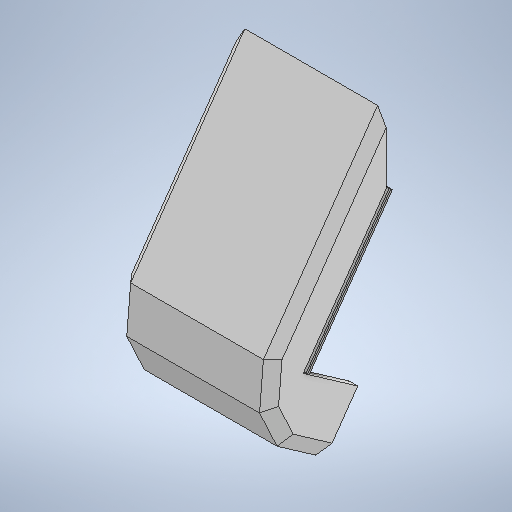
# Autodesk Inventor part: cameraholderlid v03
Saved by Autodesk Inventor 2025.2 (Build 292293000, 293)
## iProperties
Created: 2025-07-10
Part Number: cameraholderlid v03
Material: Generic
Document SubType Name: Modeling
Designer: mateo
Density: 1 g/cm^3
Appearance: Default
Author: mateo
Autodesk Inventor part; units mm, degrees
ref_plane "YZ Plane" through (0, 0, 0) normal (1, 0, 0) x (0, 1, 0)
ref_plane "XZ Plane" through (0, 0, 0) normal (0, 1, 0) x (-1, 0, 0)
ref_plane "XY Plane" through (0, 0, 0) normal (0, 0, 1) x (1, 0, 0)
sketch "Sketch1" plane through (0, 0, 0) normal (0, 0, 1) x (1, 0, 0)
  line L0 (40, -60) -> (-40, -60)
  line L1 (50, 50) -> (50, -50)
  line L2 (-50, -50) -> (-50, 50)
  line L3 (-40, 60) -> (40, 60)
  line L4 (50, -60) -> (50, 60)
  line L5 (50, 60) -> (-50, 60)
  line L6 (-50, 60) -> (-50, -60)
  line L7 (50, -60) -> (-50, -60)
  line L8 (-72, 82) -> (72, 82)
  line L9 (72, 82) -> (72, 0)
  line L10 (72, 0) -> (72, -82)
  line L11 (72, -82) -> (-72, -82)
  line L12 (-72, -82) -> (-72, 82)
  point P0 (0, 0)
  point P1 (0, 10)
  point P2 (0, 0)
  constraints: 26 end point, 3 perpendicular, 2 point on line, 1 collinear
extrude "Extrusion1" add sketch "Sketch1" along normal blind 5
sketch "Sketch2" plane through (0, 305, 5) normal (0, 0, 1) x (1, 0, 0)
  point P0 (0, 0)
  point P1 (-65, -305)
  point P2 (-65, -260)
  point P3 (-65, -350)
  point P4 (65, -305)
  point P5 (65, -260)
  point P6 (65, -350)
  point P7 (-20, -230)
  point P8 (20, -230)
  point P9 (-20, -380)
  point P10 (20, -380)
  dimension "d7" = 45
  dimension "d8" = 45
  dimension "d6" = 45
  dimension "d5" = 45
  measures "d7" distance of point (-65, -350) point (-65, -305)
  measures "d8" distance of point (-65, -305) point (-65, -260)
  measures "d6" distance of point (65, -305) point (65, -260)
  measures "d5" distance of point (65, -350) point (65, -305)
hole "Hole1" at (-65, 0, 5) at (-65, 45, 5) at (-65, -45, 5) at (65, 0, 5) at (65, 45, 5) at (65, -45, 5) at (-20, 75, 5) at (20, 75, 5) at (-20, -75, 5) at (20, -75, 5) direction (0, 0, -1) diameter 3.4587 depth 10.8 tip angle 118
move or copy body "Move Body1" bodies to move or copy 1 copy no translate (-2.5, -1.5, 0)
ref_plane "Work Plane1" through (-52.5, 58.5, 5) normal (0, -0.6427876, 0.7660444) x (1, 0, 0)
ref_plane "Work Plane2" through (47.5, -61.5, 5) normal (0, 0.5735764, 0.819152) x (-1, 0, 0)
sketch "Sketch6" plane through (47.5, -61.5, 5) normal (0, 0.5735764, 0.819152) x (-1, 0, 0)
  line L0 (102.232, 1.5875) -> (102.232, -110.9125)
  line L1 (-2.232, -110.9125) -> (-2.232, 1.5875)
  line L2 (-2.232, -110.9125) -> (102.232, -110.9125)
  line L3 (102.232, 1.5875) -> (102.232, 46.5875)
  line L4 (102.232, 46.5875) -> (-2.232, 46.5875)
  line L5 (-2.232, 46.5875) -> (-2.232, 1.5875)
  ellipse E0 centre (115, -12.2873) end of major axis (113.2706, -12.2873) minor radius 1.4166 projected
  ellipse E1 centre (-15, -12.2873) end of major axis (-16.7294, -12.2873) minor radius 1.4166 projected
  ellipse E2 centre (115, -49.1491) end of major axis (113.2706, -49.1491) minor radius 1.4166 projected
  ellipse E3 centre (-15, -49.1491) end of major axis (-16.7294, -49.1491) minor radius 1.4166 projected
  line L6 (102.232, 1.5875) -> (102.232, 46.5875)
  point P0 (47.5, -53.2457)
  dimension "d76" = 12.768
  dimension "d77" = 12.768
  dimension "d78" = 12.768
  dimension "d79" = 12.768
  constraints: 14 end point, 2 parallel, 2 perpendicular, 4 other
  measures "d76" distance from line of point (115, -12.287) L0
  measures "d77" distance from line of point (-15, -12.287) L1
  measures "d78" distance from line of L0 point (115, -49.149)
  measures "d79" distance from line of point (-15, -49.149) L1
extrude "Extrusion4" add sketch "Sketch6" along normal blind 70 contours L0 L2 L1 L5 L4 L3
sketch "Sketch8" plane through (47.5, -61.5, 5) normal (0, 0.5735764, 0.819152) x (-1, 0, 0)
  line L0 (0, -115.8875) -> (100, -115.8875) projected
  line L1 (0, -101.1661) -> (0, -2.8679) projected
  line L2 (96.232, -115.8875) -> (3.768, -115.8875)
  line L3 (102.232, 46.5875) -> (-2.232, 46.5875) projected
  line L4 (0, 46.5875) -> (100, 46.5875)
  line L5 (102.232, -110.9125) -> (102.232, -8.7172) projected
  line L6 (-2.232, -8.7172) -> (-2.232, -110.9125) projected
  line L7 (102.232, 0) -> (102.232, 46.5875) projected
  line L8 (96.232, 46.5875) -> (3.768, 46.5875)
  line L9 (3.768, 46.5875) -> (3.768, -115.8875)
  line L10 (3.768, -115.8875) -> (96.232, -115.8875)
  line L11 (96.232, -115.8875) -> (96.232, 46.5875)
  point P0 (47.5, -53.2457)
  point P1 (0, -8.7172)
  point P2 (96.232, -115.8875)
  point P3 (96.232, 46.5875)
  point P4 (3.768, 46.5875)
  point P5 (3.768, -115.8875)
  dimension "d42" = 6
  dimension "d43" = 6
  constraints: 12 end point, 2 horizontal, 2 parallel, 2 point on line, 1 perpendicular
  measures "d42" distance between parallel lines of L11 L5
  measures "d43" distance between parallel lines of L9 L6
extrude "Extrusion6" cut sketch "Sketch8" along normal blind 65
sketch "Sketch12" plane through (-54.732, -54.3593, 0) normal (-1, 0, 0) x (0, 0, 1)
  line L0 (0, 0) -> (0, 122.0413) projected
  line L1 (-1.2762, 123.8638) -> (0, 122.0413) projected
  line L2 (0, 122.0413) -> (-1.2762, 123.8638)
  line L3 (-1.2762, 123.8638) -> (-58.6698, 83.6763)
  line L4 (-58.6698, 83.6763) -> (0, -0.1129)
  line L5 (0, -0.1129) -> (0, 122.0413)
  point P0 (0, 54.3593)
  point P1 (0, 0)
  constraints: 8 end point, 2 perpendicular, 1 collinear, 1 vertical
extrude "Extrusion8" cut sketch "Sketch12" against normal through all
chamfer "Chamfer1" distance 6 angle 45 2 edges at (49.732, 0.5147, 47.0311) (-54.732, 0.5147, 47.0311)
sketch "Sketch15" plane through (47.5, -61.5, 5) normal (0, 0.5735764, 0.819152) x (-1, 0, 0)
  line L0 (96.232, -110.9125) -> (96.232, 46.5875) projected
  line L1 (3.768, -23.8125) -> (96.232, -23.8125)
  line L2 (96.232, -23.8125) -> (96.232, 11.2719)
  line L3 (3.768, 46.5875) -> (3.768, -110.9125) projected
  line L4 (3.768, 20.6375) -> (3.768, 46.5875)
  line L5 (3.768, 46.5875) -> (96.232, 46.5875)
  line L6 (96.232, 46.5875) -> (96.232, 11.2719)
  line L7 (102.232, 0) -> (102.232, 46.5875) projected
  line L8 (3.768, 46.5875) -> (3.768, -23.8125)
  point P0 (47.5, -53.2457)
  point P1 (96.6, -101.5469)
  point P2 (96.232, 46.5875)
  point P3 (2.1357, -101.5469)
  point P4 (3.768, -110.9125)
  point P5 (96.6, -100.9795)
  point P6 (2.1357, -100.9795)
  constraints: 12 end point, 1 parallel, 4 other
extrude "Extrusion11" add sketch "Sketch15" along normal blind 5 and the other way blind 3
ref_plane "Work Plane3" through (-54.732, -59.5119, 89.0621) normal (0, 0.819152, -0.5735764) x (1, 0, 0)
ref_plane "Work Plane7" through (-54.732, -84.9826, 28.6379) normal (0, 0.9786416, -0.205574) x (1, 0, 0)
sketch "Sketch28" plane through (-54.732, -84.9826, 28.6379) normal (0, 0.9786416, -0.205574) x (1, 0, 0)
  line L0 (104.464, -64.7463) -> (104.464, -63.1884) projected
  line L1 (104.464, -64.7463) -> (104.464, -63.1884)
  line L2 (98.464, -6.7829) -> (98.464, -69.7132) projected
  line L3 (104.464, -63.1884) -> (98.464, -69.7132)
  line L4 (6, -6.7829) -> (6, -69.7132) projected
  line L5 (98.464, -69.7132) -> (6, -69.7132)
  line L6 (0, -63.1884) -> (6, -69.7132) projected
  line L7 (6, -69.7132) -> (0, -63.1884)
  line L8 (0, -63.1884) -> (0, -64.7463)
  line L9 (0, -64.7463) -> (6, -70.2637)
  line L10 (6, -70.2637) -> (98.464, -70.2637)
  line L11 (98.464, -70.2637) -> (104.464, -64.7463)
  point P0 (54.732, 10.556)
  constraints: 16 end point, 3 equal length, 3 perpendicular, 1 vertical
extrude "Extrusion22" cut sketch "Sketch28" against normal through all
sketch "Sketch31" plane through (-54.732, -61.5, 5) normal (-1, 0, 0) x (0, 0, 1)
  line L0 (26.7215, -38.1622) -> (79.1472, -1.4534) projected
  line L1 (64.0809, -30.3145) -> (67.1645, -44.9941) projected
  line L2 (26.7215, -38.1622) -> (67.1645, -44.9941)
  line L3 (55.4773, -18.0272) -> (64.0809, -30.3145) projected
  line L4 (67.0706, -45.0138) -> (94.0685, -39.3427) projected
  line L5 (70.081, -44.3815) -> (67.0706, -45.0138)
  line L6 (70.081, -44.3815) -> (63.7303, -15.5115)
  line L7 (63.7303, -15.5115) -> (25.4, -18.0272)
  line L8 (25.4, -18.0272) -> (26.7215, -38.1622)
  point P0 (-5, 61.5)
  constraints: 10 end point, 1 collinear, 1 perpendicular, 1 point on line
extrude "Extrusion25" add sketch "Sketch31" against normal blind 6
sketch "Sketch32" plane through (49.732, -61.5, 5) normal (1, 0, 0) x (0, 0, -1)
  line L0 (-26.7215, -38.1622) -> (0, 0) projected
  line L1 (-26.7215, -38.1622) -> (-67.1645, -44.9941) projected
  line L2 (-26.7215, -38.1622) -> (-67.1645, -44.9941)
  line L3 (-64.0809, -30.3145) -> (-67.1645, -44.9941) projected
  line L4 (-67.1645, -44.9941) -> (-64.0809, -30.3145)
  line L5 (-55.4773, -18.0272) -> (-64.0809, -30.3145) projected
  line L6 (-64.0809, -30.3145) -> (-55.4773, -18.0272)
  line L7 (-55.4773, -18.0272) -> (-26.7215, -38.1622)
  line L8 (-67.1645, -44.9941) -> (-71.4375, -44.0965)
  line L9 (-94.0685, -39.3427) -> (-67.1656, -44.9939) projected
  line L10 (-71.4375, -44.0965) -> (-64.617, -11.6275)
  line L11 (-64.617, -11.6275) -> (-26.7215, -38.1622)
  point P0 (5, 61.5)
  constraints: 14 end point, 3 collinear, 3 perpendicular, 2 point on line
extrude "Extrusion26" add sketch "Sketch32" against normal blind 6
sketch "Sketch34" plane through (47.5, -58.6321, 9.0958) normal (0, 0.5735764, 0.819152) x (1, 0, 0)
  line L0 (-3.768, 15.858) -> (-3.768, -46.5875) projected
  line L1 (-96.232, -46.5875) -> (-96.232, 15.858) projected
  line L2 (-96.232, -46.5875) -> (-3.768, -46.5875) projected
  line L3 (-3.768, 23.8125) -> (-96.232, 23.8125) projected
  line L4 (-50, -46.5875) -> (-50, 23.8125)
  line L5 (-94, -46.5875) -> (-54, -46.5875)
  line L6 (-54, -46.5875) -> (-54, 3.4125)
  line L7 (-54, 3.4125) -> (-94, 3.4125)
  line L8 (-94, 3.4125) -> (-96.232, 3.4125)
  line L9 (-96.232, 3.4125) -> (-96.232, -46.5875)
  line L10 (-94, -46.5875) -> (-96.232, -46.5875)
  point P0 (-47.5, 53.2457)
  point P1 (-54, -46.5875)
  dimension "d100" = 92.464
  dimension "d101" = 70.4
  dimension "d112" = 50
  constraints: 14 end point, 4 perpendicular, 2 midpoint, 2 point on line, 1 horizontal, 1 parallel
  measures "d100" distance between parallel lines of L0 L1
  measures "d101" distance between parallel lines of L2 L3
  measures "d112" distance between parallel lines of L2 L7
extrude "Extrusion27" add sketch "Sketch34" along normal blind 16
sketch "Sketch35" plane through (47.5, -49.4549, 22.2022) normal (0, 0.5735764, 0.819152) x (1, 0, 0)
  circle A0 centre (-74.6125, -42.8625) radius 2
  circle A1 centre (-84.6125, -19.1625) radius 2
  line L0 (-74.6125, 141.2434) -> (-74.6125, 78.7138)
  circle A2 centre (-64.6125, -19.1625) radius 2
  line L1 (-220.5298, -133.1321) -> (71.3048, -56.0245)
  point P0 (-47.5, 53.2457)
  point P1 (-90.1769, -210.863)
  point P2 (-74.6125, -94.5783)
  point P3 (-74.6125, -94.5783)
  dimension "d115" = 4
  dimension "d117" = 4
  dimension "d121" = 50
  dimension "d122" = 20
  dimension "d123" = 23.7
  constraints: 4 end point, 3 centre point, 2 midpoint, 2 vertical alignment, 1 symmetric about line, 1 vertical, 1 other
  measures "d115" diameter of A0
  measures "d117" diameter of A1
  measures "d121" distance from line of L1 A0.centre
  measures "d122" distance of A2.centre A1.centre
  measures "d123" vertical distance of A0.centre A1.centre
extrude "Extrusion28" cut sketch "Sketch35" against normal blind 24.6695
sketch "Sketch36" plane through (-74.5, -83.5, 5) normal (0, 0, 1) x (1, 0, 0)
  line L0 (22, 22) -> (19.768, 22) projected
  line L1 (124.232, 0) -> (19.768, 0)
  line L2 (124.232, 13.701) -> (19.768, 13.701)
  line L3 (19.768, 13.701) -> (0, 13.701)
  line L4 (0, 164) -> (0, 0) projected
  line L5 (0, 13.701) -> (0, 0)
  line L6 (0, 0) -> (19.768, 0)
  line L7 (0, 0) -> (144, 0) projected
  line L8 (124.232, 13.701) -> (144, 13.701)
  line L9 (144, 0) -> (144, 164) projected
  line L10 (144, 13.701) -> (144, 0)
  line L11 (144, 0) -> (124.232, 0)
  point P0 (74.5, 83.5)
  point P1 (0, 13.701)
  constraints: 16 end point, 3 collinear, 2 point on line, 1 perpendicular
sketch "Sketch37" plane through (-49.732, -99.6622, 31.7215) normal (0, -0.819152, 0.5735764) x (1, 0, 0)
  line L0 (-5, 0) -> (99.464, 0) projected
  line L1 (0, 8) -> (0, 0)
  line L2 (94.464, 0) -> (94.4704, 0)
  line L3 (-5, 0) -> (99.464, 0) projected
  line L4 (94.4704, 0) -> (94.464, 0)
  line L5 (93.464, 0) -> (93.464, 5)
  line L6 (93.464, 0) -> (93.464, 5) projected
  line L7 (93.464, 5) -> (43.232, 5)
  line L8 (43.232, 5) -> (43.232, 21)
  line L9 (43.232, 5) -> (93.464, 5) projected
  line L10 (0, 8) -> (0, 0)
  line L11 (1, 21) -> (4.232, 21)
  line L12 (1, 8) -> (1, 21)
  line L13 (1, 29.2104) -> (1, 0) projected
  line L14 (1, -3) -> (1, 5) projected
  line L15 (0, 0) -> (0, -3)
  line L16 (93.464, -3) -> (93.464, 5) projected
  line L17 (1, -3) -> (93.464, -3)
  line L18 (93.464, -3) -> (93.464, 5)
  line L19 (1, 21) -> (43.232, 21)
  line L20 (-5, 0) -> (-5, 29.2104) projected
  line L21 (1, 21) -> (1, -3)
  line L22 (93.464, -3) -> (93.464, 5)
  line L23 (43.232, 5) -> (43.232, 21)
  point P0 (49.732, 31.1792)
  point P1 (0, 29.137)
  point P2 (1, 5)
  point P3 (0, 8)
  point P4 (93.464, 41.1414)
  point P5 (93.464, 65)
  point P6 (93.464, 35.1055)
  point P7 (1, 29.137)
  point P8 (1, 0)
  point P9 (1, 0)
  point P10 (93.464, 0)
  constraints: 30 end point, 4 vertical, 3 collinear, 3 horizontal, 3 perpendicular, 1 point on line, 10 other
extrude "Extrusion29" add sketch "Sketch37" along normal blind 15
sketch "Sketch38" plane through (-49.732, -111.9495, 40.3251) normal (0, -0.819152, 0.5735764) x (1, 0, 0)
  line L0 (3.232, 8) -> (3.232, 24) projected
  line L1 (43.232, 5) -> (43.232, 21) projected
  line L2 (3.232, 24) -> (43.232, 24)
  line L3 (43.232, 24) -> (43.232, 22.05)
  line L4 (43.232, 22.05) -> (3.232, 22.05)
  line L5 (3.232, 22.05) -> (3.232, 24)
  point P0 (49.732, 31.1792)
  point P1 (3.232, 22.05)
  dimension "d141" = 16
  constraints: 8 end point, 2 parallel, 1 horizontal, 1 perpendicular, 1 point on line
  measures "d141" distance of L0.start L0.end
extrude "Extrusion30" cut sketch "Sketch38" against normal blind 288.2125
extrude "Extrusion31" cut sketch "Sketch36" against normal blind 288.2125
sketch "Sketch40" plane through (47.5, -61.5, 5) normal (0, -0.5735764, -0.819152) x (-1, 0, 0)
  circle A0 centre (74.6125, -42.8625) radius 2 projected
  circle A1 centre (64.6125, -19.1625) radius 2 projected
  circle A2 centre (84.6125, -19.1625) radius 2 projected
  circle A3 centre (74.6125, -42.8625) radius 5.5
  circle A4 centre (84.6125, -19.1625) radius 5.5
  circle A5 centre (64.6125, -19.1625) radius 5.5
  point P0 (47.5, 53.2457)
  dimension "d136" = 11
  dimension "d137" = 11
  dimension "d138" = 11
  constraints: 3 centre point, 3 coincident
  measures "d136" diameter of A3
  measures "d137" diameter of A4
  measures "d138" diameter of A5
extrude "Extrusion32" cut sketch "Sketch40" along normal blind 3
fillet "Fillet1" radius 2 1 edges at (-2.5, -69.799, 5)
sketch "Sketch41" plane through (47.5, -58.6321, 9.0958) normal (0, 0.5735764, 0.819152) x (1, 0, 0)
  line L0 (-54, 3.4125) -> (-54, -61.5875) projected
  line L1 (22, -5.1598) -> (-122, -5.1598) projected
  line L2 (-3.768, -61.5875) -> (-54, -61.5875) projected
  circle A0 centre (-29.5, -43.75) radius 3.5
  circle A1 centre (-29.5, -15.75) radius 3.5
  point P0 (-47.5, 53.2457)
  dimension "d147" = 7
  dimension "d149" = 7
  dimension "d196" = 28
  constraints: 2 centre point
  measures "d147" diameter of A0
  measures "d149" diameter of A1
  measures "d196" distance of A1.centre A0.centre
extrude "Extrusion33" cut sketch "Sketch41" against normal through all
sketch "Sketch42" plane through (47.5, -61.5, 5) normal (0, -0.5735764, -0.819152) x (-1, 0, 0)
  line L0 (97.232, -46.5875) -> (2.768, -46.5875) projected
  arc A0 (33, -43.75) -> (33, -43.75) centre (29.5, -43.75) ccw projected
  circle A1 centre (29.5, -43.75) radius 3.5 projected
  circle A2 centre (29.5, -43.75) radius 7.5
  circle A3 centre (29.5, -15.75) radius 3.5 projected
  circle A4 centre (29.5, -15.75) radius 7.5
  point P0 (47.5, 53.2457)
  point P1 (2.768, -46.5875)
  point P2 (26, -43.75)
  point P3 (26, -43.75)
  dimension "d158" = 15
  dimension "d197" = 15
  constraints: 2 centre point, 2 coincident, 1 other
  measures "d158" diameter of A2
  measures "d197" diameter of A4
extrude "Extrusion34" cut sketch "Sketch42" along normal blind 3
sketch "Sketch44" plane through (47.5, -61.5, 5) normal (0, -0.5735764, -0.819152) x (-1, 0, 0)
  line L0 (102.232, -46.5875) -> (96.232, -46.5875) projected
  line L1 (96.232, 0) -> (96.232, -46.5875) projected
  line L2 (102.232, 0) -> (102.232, -46.5875) projected
  line L3 (100, 0) -> (102.232, 0) projected
  line L4 (96.232, 0) -> (100, 0) projected
  line L5 (100, 8.7172) -> (96.232, 8.7172) projected
  line L6 (96.232, 8.7172) -> (96.232, 0) projected
  line L7 (100, 8.7172) -> (100, 0) projected
  line L8 (96.232, 0) -> (96.232, 2.1006) projected
  line L9 (102.232, -46.5875) -> (96.232, -46.5875)
  line L10 (96.232, -46.5875) -> (96.232, 0)
  line L11 (96.232, 0) -> (102.232, 0)
  line L12 (102.232, 0) -> (102.232, -46.5875)
  line L13 (3.768, -46.5875) -> (3.768, 0) projected
  line L14 (0, 0) -> (3.768, 0) projected
  line L15 (-2.232, 0) -> (0, 0) projected
  line L16 (-2.232, -46.5875) -> (-2.232, 0) projected
  line L17 (3.768, 8.7172) -> (0, 8.7172) projected
  line L18 (0, 0) -> (0, 8.7172) projected
  line L19 (3.768, 0) -> (3.768, 8.7172) projected
  line L20 (2.768, -46.5875) -> (-2.232, -46.5875)
  line L21 (-2.232, -46.5875) -> (-2.232, 0)
  line L22 (-2.232, 0) -> (2.768, 0)
  line L23 (2.768, 0) -> (2.768, -46.5875)
  line L24 (96.232, 0) -> (100, 0) projected
  line L25 (102.232, -46.5875) -> (96.232, -46.5875)
  line L26 (96.232, -46.5875) -> (96.232, 0)
  line L27 (96.232, 0) -> (102.232, 0)
  line L28 (102.232, 0) -> (102.232, -46.5875)
  line L29 (-2.232, -46.5875) -> (-2.232, 0) projected
  line L30 (2.768, -46.5875) -> (-2.232, -46.5875)
  line L31 (-2.232, -46.5875) -> (-2.232, 0)
  line L32 (-2.232, 0) -> (2.768, 0)
  line L33 (2.768, 0) -> (2.768, -46.5875)
  line L34 (96.232, 0) -> (96.232, -46.5875) projected
  line L35 (102.232, 0) -> (102.232, -46.5875) projected
  line L36 (100, 0) -> (102.232, 0) projected
  line L37 (96.232, 0) -> (100, 0) projected
  line L38 (102.232, -46.5875) -> (96.232, -46.5875) projected
  line L39 (3.768, -46.5875) -> (-2.232, -46.5875) projected
  line L40 (100, 8.7172) -> (96.232, 8.7172) projected
  line L41 (96.232, 8.7172) -> (96.232, 0) projected
  line L42 (100, 8.7172) -> (100, 0) projected
  line L43 (3.768, -46.5875) -> (3.768, 0) projected
  line L44 (0, 0) -> (3.768, 0) projected
  line L45 (-2.232, 0) -> (0, 0) projected
  line L46 (-2.232, -46.5875) -> (-2.232, 0) projected
  line L47 (102.232, -46.5875) -> (96.232, -46.5875) projected
  line L48 (3.768, -46.5875) -> (-2.232, -46.5875) projected
  line L49 (3.768, 8.7172) -> (0, 8.7172) projected
  line L50 (0, 0) -> (0, 8.7172) projected
  line L51 (3.768, 0) -> (3.768, 8.7172) projected
  point P0 (47.5, 53.2457)
  point P1 (102.232, -46.5875)
  point P2 (2.768, 0)
  constraints: 32 end point, 8 parallel, 4 horizontal, 4 perpendicular
extrude "Extrusion35" add sketch "Sketch44" along normal blind 3 contours L0 L1 L4 L3 L2 | L39 L23 L14 L13 | L20 L16 L15 L14 L23
ref_plane "Work Plane8" through (44.732, -106.4941, 72.1645) normal (0, -0.9860303, -0.166566) x (1, 0, 0)
sketch "Sketch45" plane through (44.732, -106.4941, 72.1645) normal (0, -0.9860303, -0.166566) x (1, 0, 0)
  line L0 (-99.464, -41.016) -> (-99.464, 0) projected
  line L1 (-99.464, -41.016) -> (5, -41.016) projected
  line L2 (5, 0) -> (5, -41.016) projected
  line L3 (-1, -33.9952) -> (-1, 0) projected
  line L4 (-1, -41.016) -> (5, -41.016) projected
  line L5 (-99.464, 0) -> (-93.464, 0)
  line L6 (-99.464, -41.016) -> (-99.464, 0)
  line L7 (5, 0) -> (5, -41.016) projected
  line L8 (0, 0) -> (5, 0)
  line L9 (5, 0) -> (5, -41.016)
  line L10 (-1, -41.016) -> (-1, -33.9952) projected
  line L11 (5, -72.8496) -> (5, -43.1525) projected
  line L12 (5, -43.1525) -> (-99.464, -43.1525) projected
  line L13 (5, -43.1525) -> (-1, -43.1525)
  line L14 (-1, -43.1525) -> (-1, 0)
  line L15 (5, 0) -> (5, -43.1525)
  line L16 (5, -43.1525) -> (-99.464, -43.1525) projected
  line L17 (-99.464, -41.016) -> (-99.464, -43.1525)
  line L18 (-99.464, -43.1525) -> (-93.464, -43.1525)
  line L19 (-93.464, -43.1525) -> (-93.464, -41.016)
  line L20 (-93.464, 0) -> (-99.464, 0)
  line L21 (-99.464, 0) -> (-99.464, -43.1525)
  line L22 (-99.464, -43.1525) -> (-93.464, -43.1525)
  line L23 (-93.464, 0) -> (-93.464, -43.1525)
  line L24 (-93.464, -98.7163) -> (-93.464, 15.8051) projected
  line L25 (5, 0) -> (-1, 0) projected
  point P0 (-44.732, -88.8947)
  point P1 (-94.464, -0.1031)
  point P2 (-94.464, -41.016)
  point P3 (-93.464, -0.1031)
  point P4 (5, -41.016)
  point P5 (-1, -41.016)
  point P6 (-93.464, -41.016)
  point P7 (-99.464, -41.016)
  constraints: 28 end point, 7 collinear, 3 horizontal, 1 perpendicular, 1 vertical
extrude "Extrusion37" add sketch "Sketch45" along normal blind 15 contours L0 L5 L23 L1 | L1 L19 L12 L17 | L1 L15 L12 L14
sketch "Sketch47" plane through (49.732, -66.7303, 5) normal (1, 0, 0) x (0, 0, -1)
  line L0 (-67.0629, -39.7466) -> (-67.0706, -39.7835) projected
  line L1 (-67.0706, -39.7835) -> (-27.0245, -48.1956)
  line L2 (-64.6661, -54.5542) -> (-22.1163, -47.3665) projected
  line L3 (-27.0245, -48.1956) -> (-64.578, -54.5394)
  line L4 (-67.1645, -39.7638) -> (-94.0685, -34.1123) projected
  line L5 (-64.578, -54.5394) -> (-64.6661, -54.5542)
  line L6 (-67.1645, -39.7638) -> (-64.6661, -54.5542) projected
  line L7 (-67.1645, -39.7638) -> (-67.0706, -39.7835)
  point P0 (5, 66.7303)
  point P1 (-32.8677, -46.9399)
  point P2 (-24.223, -47.7224)
  point P3 (-63.9955, -25.144)
  constraints: 8 end point, 2 collinear, 1 point on line
extrude "Extrusion38" cut sketch "Sketch47" against normal blind 120
sketch "Sketch49" plane through (-48.732, -54.3593, 0) normal (-1, 0, 0) x (0, 0, 1)
  line L0 (0, 8.7172) -> (44.4209, -54.7224) projected
  line L1 (0, 8.7172) -> (0, -5.2303)
  line L2 (1.3377, -7.1407) -> (-11.1157, 10.6446) projected
  line L3 (-11.1157, 10.6446) -> (-4.3813, 15.3601)
  line L4 (-4.3813, 15.3601) -> (0, 8.7172)
  line L5 (0, 8.7172) -> (-4.5625, 15.2332) projected
  line L6 (-11.1157, 10.6446) -> (0, -5.2303)
  point P0 (0, 54.3593)
  constraints: 8 end point, 3 point on line, 2 perpendicular, 1 vertical
extrude "Extrusion40" cut sketch "Sketch49" against normal through all contours L1 L2 L3 L5
sketch "Sketch50" plane through (-48.732, -55.8368, 7.1384) normal (0, 0.819152, -0.5735764) x (1, 0, 0)
  line L0 (42.232, -16) -> (0, -16) projected
  line L1 (9.0575, -16) -> (7.9375, -16)
  arc A0 (34.925, -16) -> (9.0575, -16) centre (21.9913, -30.5193) ccw
  line L2 (34.925, -16) -> (9.0575, -16)
  point P0 (48.732, -26.1792)
  point P1 (33.6195, -16)
  point P2 (9.0575, -16)
  constraints: 4 end point, 2 point on circle, 2 point on line, 1 centre point
extrude "Extrusion41" cut sketch "Sketch50" against normal blind 18.575
sketch "Sketch52" plane through (-54.732, -66.7303, 5) normal (-1, 0, 0) x (0, 0, 1)
  line L0 (26.7215, -32.9319) -> (24.223, -47.7224) projected
  line L1 (27.0245, -48.1956) -> (94.0685, -34.1123) projected
  line L2 (24.223, -47.7224) -> (27.0245, -48.1956) projected
  line L3 (32.8677, -46.9399) -> (26.0097, -37.1457) projected
  line L4 (26.0097, -37.1457) -> (32.8677, -46.9399)
  line L5 (27.0245, -48.1956) -> (24.223, -47.7224)
  line L6 (26.0097, -37.1457) -> (24.223, -47.7224)
  line L7 (32.8677, -46.9399) -> (32.9391, -47.042)
  line L8 (32.9391, -47.042) -> (27.0245, -48.1956)
  point P0 (-5, 66.7303)
  point P1 (32.8849, -46.9646)
  constraints: 10 end point, 2 collinear, 1 perpendicular, 1 point on line
extrude "Extrusion43" cut sketch "Sketch52" against normal through all contours L3 L7 L1 L2 L0
sketch "Sketch53" plane through (-54.732, -66.7303, 5) normal (-1, 0, 0) x (0, 0, 1)
  line L0 (0, 116.8109) -> (85.4767, -5.2624) projected
  line L1 (12.7, 98.6735) -> (85.4767, -5.2624)
  line L2 (12.7, 81.631) -> (12.7, 130.812)
  line L3 (12.7, 130.812) -> (12.7, 81.631)
  line L4 (12.7, 81.631) -> (12.7, 61.9125)
  line L5 (12.7, 61.9125) -> (102.0312, -65.6657)
  line L6 (12.7, 130.812) -> (-12.7, 180.975)
  line L7 (-12.7, 180.975) -> (-12.7, -92.075)
  line L8 (-12.7, -92.075) -> (102.0312, -65.6657)
  point P0 (-5, 66.7303)
  point P1 (87.7509, -8.5103)
  dimension "d233" = 145
  constraints: 16 end point, 2 point on line, 2 vertical, 1 collinear
  measures "d233" angle of L5 L4
extrude "Extrusion44" cut sketch "Sketch53" against normal through all
sketch "Sketch56" plane through (-54.732, -66.7303, 5) normal (-1, 0, 0) x (0, 0, 1)
  line L0 (24.264, -34.6526) -> (22.1163, -47.3665) projected
  line L1 (24.223, -47.7224) -> (26.0097, -37.1457) projected
  line L2 (24.264, -34.6526) -> (26.0097, -37.1457)
  line L3 (26.0097, -37.1457) -> (24.223, -47.7224)
  line L4 (24.223, -47.7224) -> (21.9676, -47.3414)
  line L5 (21.9676, -47.3414) -> (24.264, -34.6526)
  point P0 (-5, 66.7303)
  constraints: 8 end point, 1 collinear, 1 perpendicular
extrude "Extrusion46" cut sketch "Sketch56" against normal through all contours L2 L1 L4 L0
sketch "Sketch59" plane through (69.5, 80.5, 0) normal (0, 0, -1) x (-1, 0, 0)
  line L0 (124.232, -148.2248) -> (124.232, -65.5994) projected
  line L1 (124.232, -131.7625) -> (22.225, -131.7625)
  line L2 (22.225, -144.4625) -> (124.232, -144.4625)
  line L3 (124.232, -144.4625) -> (124.232, -131.7625)
  line L4 (22.225, -144.4625) -> (19.05, -144.4625)
  line L5 (19.05, -144.4625) -> (19.05, -131.7625)
  line L6 (19.05, -131.7625) -> (22.225, -131.7625)
  point P0 (69.5, -80.5)
  point P1 (22.225, -131.7625)
  constraints: 12 end point, 2 horizontal, 2 parallel, 1 perpendicular, 1 point on line
extrude "Extrusion48" add sketch "Sketch59" against normal blind 1
sketch "Sketch60" plane through (-74.5, 80.5, 0) normal (-1, 0, 0) x (0, 0, 1)
  line L0 (17.4625, 4.7625) -> (-19.05, 4.7625)
  line L1 (-19.05, 4.7625) -> (-19.05, -168.275)
  line L2 (-19.05, -168.275) -> (17.4625, -168.275)
  line L3 (17.4625, -168.275) -> (17.4625, 4.7625)
  point P0 (0, -80.5)
  constraints: 8 end point, 2 parallel, 1 horizontal, 1 perpendicular
extrude "Extrusion50" cut sketch "Sketch60" against normal through all
sketch "Sketch61" plane through (49.732, -4.8178, 17.7) normal (1, 0, 0) x (0, 0, -1)
  line L0 (-49.1752, -70.2295) -> (-66.4472, -58.1355) projected
  line L1 (-51.9844, -68.2625) -> (-49.1752, -70.2295)
  line L2 (-53.6682, -76.6461) -> (-51.917, -68.3097) projected
  line L3 (-54.6484, -78.4401) -> (-51.917, -68.3097)
  line L4 (-54.6484, -78.4401) -> (-47.625, -71.4375)
  line L5 (-49.1752, -70.2295) -> (-47.625, -71.4375)
  line L6 (-49.1752, -70.2295) -> (-51.917, -68.3097)
  point P0 (17.7, 4.8178)
  constraints: 10 end point, 2 collinear, 1 point on line
extrude "Extrusion51" cut sketch "Sketch61" against normal blind 149.7
sketch "Sketch62" plane through (-48.732, -62.3798, 84.9664) normal (0, -0.819152, 0.5735764) x (1, 0, 0)
  line L0 (-6, -22.0852) -> (0, -22.0852) projected
  line L1 (-2, -22.0852) -> (-2, -27.0852)
  line L2 (-4, -27.0852) -> (-4, -22.0852)
  line L3 (-6, -22.0852) -> (-6, -29.1506)
  line L4 (-1, -28.5852) -> (-5, -28.5852)
  line L5 (-5, -28.5852) -> (-5, -27.0852)
  line L6 (-1, -28.5852) -> (-1, -27.0852)
  line L7 (0, -22.0852) -> (0, -28.5852)
  line L8 (-4, -22.0852) -> (-4, -22.0852)
  line L9 (-6, -22.0852) -> (0, -22.0852) projected
  line L10 (-2, -22.0852) -> (-2, -22.0852)
  line L11 (-5, -27.0852) -> (-4, -27.0852)
  line L12 (-2, -27.0852) -> (-1, -27.0852)
  line L13 (-6, -22.0852) -> (-6, -1) projected
  line L14 (-6, -11.5426) -> (46.232, -11.5426)
  line L15 (46.232, -11.5426) -> (46.232, 19.05)
  line L16 (46.232, 19.05) -> (46.232, -31.75)
  line L17 (94.464, -22.0852) -> (94.464, -27.0852)
  line L18 (96.464, -27.0852) -> (96.464, -22.0852)
  line L19 (93.464, -28.5852) -> (97.464, -28.5852)
  line L20 (97.464, -28.5852) -> (97.464, -27.0852)
  line L21 (93.464, -28.5852) -> (93.464, -27.0852)
  line L22 (97.464, -27.0852) -> (96.464, -27.0852)
  line L23 (94.464, -27.0852) -> (93.464, -27.0852)
  line L24 (94.464, -22.0852) -> (94.464, -22.0432)
  line L25 (94.464, -22.0432) -> (96.464, -22.0432)
  line L26 (98.464, -22.0852) -> (92.464, -22.0852) projected
  line L27 (96.464, -22.0432) -> (96.464, -22.0852)
  point P0 (48.732, -33.8208)
  point P1 (0, -25.3352)
  point P2 (-2, -22.0852)
  dimension "d226" = 2
  dimension "d227" = 1.5
  dimension "d228" = 1
  dimension "d229" = 1
  dimension "d230" = 2
  dimension "d236" = 52.232
  constraints: 48 end point, 8 symmetric about line, 5 vertical, 4 parallel, 4 point on line, 3 horizontal, 3 perpendicular, 2 midpoint, 1 collinear
  measures "d226" distance between parallel lines of L2 L3
  measures "d227" distance of L4.end L5.end
  measures "d228" distance between parallel lines of L7 L6
  measures "d229" distance between parallel lines of L3 L5
  measures "d230" distance from line of point (0, -25.335) L1
  measures "d236" distance of L14.start L14.end
extrude "Extrusion52" add sketch "Sketch62" against normal up to surface (85.7344 mm away)
sketch "Sketch63" plane through (-48.732, -62.3798, 84.9664) normal (0, -0.819152, 0.5735764) x (1, 0, 0)
  line L0 (-6, -22.0852) -> (-6, -1) projected
  line L1 (-6, -1) -> (-6, -22.0852) projected
  line L2 (-6, -22.0852) -> (-6, -1)
  line L3 (-6, -1) -> (0, 5) projected
  line L4 (-6, -1) -> (0, 5)
  line L5 (0, 5) -> (92.464, 5)
  line L6 (92.464, 5) -> (98.464, -1)
  line L7 (98.464, -1) -> (98.464, -22.0852)
  line L8 (92.464, 0) -> (92.464, -22.0852) projected
  line L9 (92.464, -22.0852) -> (92.464, 0)
  line L10 (92.464, 0) -> (0, 0)
  line L11 (0, 0) -> (0, -21.358)
  line L12 (-2, -22.0852) -> (0, -22.0852) projected
  line L13 (0, -22.0852) -> (0, -21.358)
  line L14 (0, -22.0852) -> (0, 0) projected
  line L15 (-6, -22.0852) -> (-4, -22.0852) projected
  line L16 (-4, -27.0852) -> (-4, -22.0852) projected
  line L17 (-4, -22.0852) -> (-4, -27.0852)
  line L18 (-5, -27.0852) -> (-5, -28.5852) projected
  line L19 (0, -22.0852) -> (0, 0) projected
  line L20 (0, 0) -> (92.464, 0) projected
  line L21 (92.464, 0) -> (92.464, -22.0852) projected
  line L22 (98.464, -22.0852) -> (96.464, -22.0852) projected
  line L23 (98.464, -22.0852) -> (98.464, -1) projected
  line L24 (92.464, 5) -> (98.464, -1) projected
  line L25 (0, 5) -> (92.464, 5) projected
  line L26 (-6, -1) -> (0, 5) projected
  line L27 (-6, -22.0852) -> (-6, -1) projected
  line L28 (-6, -22.0852) -> (-4, -22.0852) projected
  line L29 (-4, -22.0852) -> (-4, -27.0852) projected
  line L30 (-4, -27.0852) -> (-5, -27.0852) projected
  line L31 (-5, -27.0852) -> (-5, -28.5852) projected
  line L32 (-5, -28.5852) -> (-1, -28.5852) projected
  line L33 (-1, -28.5852) -> (-1, -27.0852) projected
  line L34 (-1, -27.0852) -> (-2, -27.0852) projected
  line L35 (-2, -27.0852) -> (-2, -22.0852) projected
  line L36 (-2, -22.0852) -> (0, -22.0852) projected
  line L37 (-4, -27.0852) -> (-5, -27.0852) projected
  line L38 (-4, -27.0852) -> (-5, -27.0852)
  line L39 (-5, -28.5852) -> (-5, -27.0852) projected
  line L40 (-5, -27.0852) -> (-5, -28.5852)
  line L41 (-5, -28.5852) -> (-1, -28.5852) projected
  line L42 (-5, -28.5852) -> (-1, -28.5852)
  line L43 (-1, -28.5852) -> (-1, -27.0852)
  line L44 (-2, -27.0852) -> (-2, -22.0852)
  line L45 (0, -22.0852) -> (-2, -22.0852)
  line L46 (-4, -22.0852) -> (-6, -22.0852)
  line L47 (94.464, -22.0852) -> (92.464, -22.0852) projected
  line L48 (94.464, -22.0852) -> (94.464, -27.0852) projected
  line L49 (94.464, -27.0852) -> (93.464, -27.0852) projected
  line L50 (93.464, -27.0852) -> (93.464, -28.5852) projected
  line L51 (93.464, -28.5852) -> (97.464, -28.5852) projected
  line L52 (97.464, -28.5852) -> (97.464, -27.0852) projected
  line L53 (97.464, -27.0852) -> (96.464, -27.0852) projected
  line L54 (96.464, -27.0852) -> (96.464, -22.0852) projected
  line L55 (96.464, -22.0852) -> (96.464, -27.0852)
  line L56 (97.464, -27.0852) -> (97.464, -28.5852)
  line L57 (96.464, -27.0852) -> (97.464, -27.0852)
  line L58 (97.464, -28.5852) -> (93.464, -28.5852)
  line L59 (93.464, -27.0852) -> (94.464, -27.0852)
  line L60 (94.464, -27.0852) -> (94.464, -22.0852)
  line L61 (93.464, -28.5852) -> (93.464, -27.0852)
  point P0 (48.732, -33.8208)
  point P1 (-2, -22.0852)
  point P2 (-4, -27.0852)
  point P3 (-5, -27.0852)
  point P4 (-5, -28.5852)
  constraints: 49 end point, 9 collinear, 7 perpendicular, 1 parallel
extrude "Extrusion53" add sketch "Sketch63" along normal blind 15.03
ref_plane "Work Plane9" through (-53.732, -91.0874, 70.1716) normal (0, -0.9961947, 0.0871557) x (1, 0, 0)
sketch "Sketch65" plane through (-53.732, -91.0874, 70.1716) normal (0, -0.9961947, 0.0871557) x (1, 0, 0)
  line L0 (5, 5.6292) -> (5, 24.7555) projected
  line L1 (3, 5.6292) -> (5, 5.6292) projected
  line L2 (-1, 23.8895) -> (-1, 5.6292) projected
  line L3 (-1, 5.6292) -> (1, 5.6292) projected
  line L4 (99.464, 5.6292) -> (99.464, 1.299) projected
  line L5 (99.464, 1.299) -> (98.464, 1.299) projected
  line L6 (98.464, 1.299) -> (98.464, 0) projected
  line L7 (98.464, 0) -> (102.464, 0) projected
  line L8 (102.464, 0) -> (102.464, 1.299) projected
  line L9 (102.464, 1.299) -> (101.464, 1.299) projected
  line L10 (101.464, 1.299) -> (101.464, 5.6292) projected
  line L11 (101.464, 5.6292) -> (103.464, 5.6292) projected
  line L12 (103.464, 5.6292) -> (103.464, 23.8895) projected
  line L13 (103.464, 23.8895) -> (97.464, 29.0857) projected
  line L14 (97.464, 29.0857) -> (5, 29.0857) projected
  line L15 (5, 29.0857) -> (-1, 23.8895) projected
  line L16 (-1, 23.8895) -> (-1, 5.6292) projected
  line L17 (-1, 5.6292) -> (1, 5.6292) projected
  line L18 (1, 5.6292) -> (1, 1.299) projected
  line L19 (1, 1.299) -> (0, 1.299) projected
  line L20 (0, 1.299) -> (0, 0) projected
  line L21 (0, 0) -> (4, 0) projected
  line L22 (4, 0) -> (4, 1.299) projected
  line L23 (4, 1.299) -> (3, 1.299) projected
  line L24 (3, 1.299) -> (3, 5.6292) projected
  line L25 (3, 5.6292) -> (5, 5.6292) projected
  line L26 (5, 5.6292) -> (5, 24.7555) projected
  line L27 (5, 24.7555) -> (97.464, 24.7555) projected
  line L28 (97.464, 24.7555) -> (97.464, 5.6292) projected
  line L29 (97.464, 5.6292) -> (99.464, 5.6292) projected
  line L30 (-1, 5.6292) -> (5, 5.6292)
  line L31 (5, 5.6292) -> (5, 24.7555)
  line L32 (5, 24.7555) -> (97.464, 24.7555)
  line L33 (97.464, 24.7555) -> (97.464, 5.6292)
  line L34 (97.464, 5.6292) -> (103.464, 5.6292)
  line L35 (103.464, 23.8895) -> (103.464, -41.5491) projected
  line L36 (103.464, 5.6292) -> (103.464, 23.8895)
  line L37 (103.464, 23.8895) -> (97.464, 29.0857)
  line L38 (97.464, 29.0857) -> (5, 29.0857)
  line L39 (5, 29.0857) -> (-1, 23.8895)
  line L40 (-1, 23.8895) -> (-1, 5.6292)
  point P0 (53.732, -61.9658)
  constraints: 20 end point, 5 collinear, 2 perpendicular, 1 horizontal, 1 vertical
extrude "Extrusion55" add sketch "Sketch65" along normal mid plane 35 contours L1 L30 L3 L2 L15 L14 L13 L12 L11 L34 L29 L28 L27 L0
sketch "Sketch67" plane through (-53.732, -73.654, 68.6464) normal (0, 0.9961947, -0.0871557) x (1, 0, 0)
  line L0 (97.464, -28.6772) -> (103.464, -21.749) projected
  line L1 (103.464, -23.8895) -> (103.464, -21.749) projected
  line L2 (103.464, -23.8895) -> (103.464, -21.749)
  line L3 (97.464, 40.6374) -> (97.464, -28.6772) projected
  line L4 (103.464, -21.749) -> (97.464, -28.6772)
  line L5 (5, 40.6374) -> (5, -28.6772) projected
  line L6 (97.464, -28.6772) -> (5, -28.6772)
  line L7 (-1, -21.749) -> (-1, -23.8895) projected
  line L8 (5, -28.6772) -> (-1, -21.749)
  line L9 (-1, -21.749) -> (-1, -23.8895)
  line L10 (-1, -23.8895) -> (5, -29.0857)
  line L11 (5, -29.0857) -> (97.464, -29.0857)
  line L12 (97.464, -29.0857) -> (103.464, -23.8895)
  point P0 (53.732, 61.9658)
  constraints: 16 end point, 4 equal length, 3 perpendicular
extrude "Extrusion56" cut sketch "Sketch67" against normal through all
ref_plane "Work Plane10" through (-54.732, -108.0302, 77.3046) normal (0, -0.9063078, -0.4226183) x (1, 0, 0)
sketch "Sketch68" plane through (-54.732, -108.0302, 77.3046) normal (0, -0.9063078, -0.4226183) x (1, 0, 0)
  line L0 (0, 13.9602) -> (0, 0) projected
  line L1 (6, 19.9602) -> (0, 13.9602) projected
  line L2 (0, 13.9602) -> (0, 0) projected
  line L3 (0, 0) -> (6, 0) projected
  line L4 (6, 0) -> (6, 16.5639) projected
  line L5 (6, 16.5639) -> (98.464, 16.5639) projected
  line L6 (98.464, 16.5639) -> (98.464, 0) projected
  line L7 (98.464, 0) -> (104.464, 0) projected
  line L8 (104.464, 0) -> (104.464, 13.9602) projected
  line L9 (104.464, 13.9602) -> (98.464, 19.9602) projected
  line L10 (98.464, 19.9602) -> (6, 19.9602) projected
  line L11 (0, 0) -> (6, 0) projected
  line L12 (6, 0) -> (0, 0)
  line L13 (0, 0) -> (0, 13.9602)
  line L14 (0, 13.9602) -> (6, 19.9602)
  line L15 (6, 19.9602) -> (98.464, 19.9602)
  line L16 (98.464, 19.9602) -> (104.464, 13.9602)
  line L17 (104.464, 0) -> (104.464, 13.9602) projected
  line L18 (104.464, 13.9602) -> (104.464, 0)
  line L19 (104.464, 0) -> (98.464, 0)
  line L20 (98.464, 0) -> (98.464, 16.5639)
  line L21 (98.464, 16.5639) -> (6, 16.5639)
  line L22 (6, 16.5639) -> (6, 0)
  line L23 (6, 16.5639) -> (98.464, 16.5639)
  line L24 (98.464, 16.5639) -> (98.464, 14.5516)
  line L25 (98.464, 14.5516) -> (6, 14.5516)
  line L26 (6, 14.5516) -> (6, 16.5639)
  point P0 (54.732, -115.7173)
  point P1 (6, 14.5516)
  point P2 (98.464, 14.5516)
  constraints: 29 end point, 6 equal length, 3 perpendicular, 2 horizontal, 2 point on line
extrude "Extrusion57" add sketch "Sketch68" along normal mid plane 30
ref_plane "Work Plane11" through (-54.732, -121.6249, 70.9653) normal (0, -0.5735764, -0.819152) x (1, 0, 0)
sketch "Sketch69" plane through (-54.732, -94.4356, 83.6438) normal (0, 0.9063078, 0.4226183) x (1, 0, 0)
  line L0 (104.464, 3.5398) -> (104.464, -9.9534) projected
  line L1 (104.464, -13.9602) -> (104.464, -9.9534) projected
  line L2 (104.464, -9.9534) -> (104.464, -13.9602)
  line L3 (98.464, -19.9602) -> (104.464, -13.9602) projected
  line L4 (104.464, -13.9602) -> (98.464, -19.9602)
  line L5 (98.464, -19.9602) -> (6, -19.9602)
  line L6 (6, -17.9534) -> (98.464, -17.9534) projected
  line L7 (6, -19.9602) -> (0, -13.9602)
  line L8 (0, -13.9602) -> (0, -9.9534)
  line L9 (0, -9.9534) -> (6, -17.9534) projected
  line L10 (0, -9.9534) -> (6, -17.9534)
  line L11 (6, -17.9534) -> (98.464, -17.9534)
  line L12 (98.464, -17.9534) -> (104.464, -9.9534) projected
  line L13 (98.464, -17.9534) -> (104.464, -9.9534)
  point P0 (54.732, 115.7173)
  constraints: 16 end point, 7 equal length, 1 perpendicular
extrude "Extrusion58" cut sketch "Sketch69" against normal through all
sketch "Sketch70" plane through (-54.732, -121.6249, 70.9653) normal (0, -0.5735764, -0.819152) x (1, 0, 0)
  line L0 (6, 15.5481) -> (0, 8.6199) projected
  line L1 (0, 8.6199) -> (0, 0) projected
  line L2 (0, 0) -> (6, 0) projected
  line L3 (6, 0) -> (6, 12.6021) projected
  line L4 (98.464, 12.6021) -> (98.464, 0) projected
  line L5 (98.464, 0) -> (104.464, 0) projected
  line L6 (104.464, 0) -> (104.464, 8.6199) projected
  line L7 (104.464, 8.6199) -> (98.464, 15.5481) projected
  line L8 (98.464, 15.5481) -> (6, 15.5481) projected
  line L9 (6, 12.6021) -> (98.464, 12.6021) projected
  line L10 (6, 12.6021) -> (98.464, 12.6021)
  line L11 (98.464, 12.6021) -> (98.464, 9.5481)
  line L12 (98.464, 9.5481) -> (6, 9.5481)
  line L13 (6, 9.5481) -> (6, 12.6021)
  point P0 (54.732, -140.3333)
  point P1 (6, 9.5481)
  dimension "d259" = 6
  constraints: 8 end point, 2 parallel, 1 horizontal, 1 perpendicular, 1 point on line
  measures "d259" distance between parallel lines of L12 L8
extrude "Extrusion59" add sketch "Sketch70" along normal mid plane 20
sketch "Sketch71" plane through (-54.732, -115.8891, 79.1568) normal (0, 0.5735764, 0.819152) x (1, 0, 0)
  line L0 (98.464, -14.9573) -> (104.464, -5.7197) projected
  line L1 (6, -14.9573) -> (98.464, -14.9573) projected
  line L2 (0, -5.7197) -> (6, -14.9573) projected
  line L3 (0, -5.7197) -> (0, -8.6199) projected
  line L4 (0, -8.6199) -> (6, -15.5481) projected
  line L5 (6, -15.5481) -> (98.464, -15.5481) projected
  line L6 (98.464, -15.5481) -> (104.464, -8.6199) projected
  line L7 (104.464, -8.6199) -> (104.464, -5.7197) projected
  point P0 (54.732, 140.3333)
extrude "Extrusion60" cut sketch "Sketch71" against normal through all
sketch "Sketch72" plane through (-54.732, -4.8178, 17.7) normal (-1, 0, 0) x (0, 0, 1)
  line L0 (45.0738, -122.5428) -> (48.3544, -127.228) projected
  line L1 (45.0738, -122.5428) -> (30.4648, -101.6789)
  line L2 (57.7961, -82.5414) -> (59.6046, -103.2124) projected
  line L3 (57.7961, -82.5414) -> (30.4648, -101.6789)
  line L4 (59.6046, -103.2124) -> (53.2653, -116.807) projected
  line L5 (57.7961, -82.5414) -> (59.6046, -103.2124)
  line L6 (59.6046, -103.2124) -> (53.2653, -116.807) projected
  line L7 (53.2653, -116.807) -> (45.0738, -122.5428) projected
  point P0 (-17.7, 4.8178)
  constraints: 6 end point, 1 collinear, 1 perpendicular
extrude "Extrusion61" add sketch "Sketch72" against normal blind 6
sketch "Sketch73" plane through (49.732, -4.8178, 17.7) normal (1, 0, 0) x (0, 0, -1)
  line L0 (-50.5503, -130.3641) -> (-30.4648, -101.6789) projected
  line L1 (-30.4648, -101.6789) -> (-57.7961, -82.5414) projected
  line L2 (-59.6046, -103.2124) -> (-53.2653, -116.807) projected
  line L3 (-53.2653, -116.807) -> (-45.0738, -122.5428) projected
  line L4 (-57.7961, -82.5414) -> (-59.6046, -103.2124) projected
  point P0 (17.7, 4.8178)
  point P1 (-52.302, -132.8658)
extrude "Extrusion62" add sketch "Sketch73" against normal blind 6
sketch "Sketch74" plane through (-54.732, -127.3606, 62.7738) normal (0, -0.5735764, -0.819152) x (-1, 0, 0)
  line L0 (-6, -14.9573) -> (0, -5.7197) projected
  line L1 (0, -5.7197) -> (0, 25.47) projected
  line L2 (0, 25.47) -> (-6, 25.47) projected
  line L3 (-6, -9.5481) -> (-6, 25.47) projected
  line L4 (-6, -9.5481) -> (-98.464, -9.5481) projected
  line L5 (-98.464, -9.5481) -> (-98.464, 25.47) projected
  line L6 (-104.464, 25.47) -> (-98.464, 25.47) projected
  line L7 (-104.464, -5.7197) -> (-104.464, 25.47) projected
  line L8 (-104.464, -5.7197) -> (-98.464, -14.9573) projected
  line L9 (-98.464, -14.9573) -> (-6, -14.9573) projected
  point P0 (-54.732, 140.3333)
extrude "Extrusion63" add sketch "Sketch74" along normal blind 13
body "Solid1"
